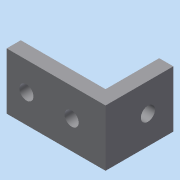
# Autodesk Inventor part: corner bracket
Saved by Autodesk Inventor 2015 (Build 190159000, 159)
## iProperties
Created: 2016-09-09
Part Number: corner bracket
Material: Generic
Document SubType Name: Modeling
Designer: Dustin
Density: 1 g/cm^3
Appearance: Default
Author: Dustin
Autodesk Inventor part; units mm, degrees
ref_plane "YZ Plane" through (0, 0, 0) normal (1, 0, 0) x (0, 1, 0)
ref_plane "XZ Plane" through (0, 0, 0) normal (0, 1, 0) x (-1, 0, 0)
ref_plane "XY Plane" through (0, 0, 0) normal (0, 0, 1) x (1, 0, 0)
sketch "Sketch1" plane through (0, 0, 0) normal (0, 0, 1) x (1, 0, 0)
  line L0 (0, 0) -> (35, 0)
  line L1 (35, 0) -> (35, 5)
  line L2 (35, 5) -> (0, 5)
  line L3 (0, 5) -> (0, 0)
  line L4 (35, 5) -> (30, 5)
  line L5 (30, 5) -> (30, 24)
  line L6 (30, 24) -> (35, 24)
  line L7 (35, 24) -> (35, 5)
  dimension "d0" = 5
  dimension "d1" = 5
  dimension "d2" = 35
  dimension "d3" = 19
  constraints: 16 end point, 4 parallel, 2 horizontal, 2 perpendicular
  measures "d0" distance of L2.end L0.start
  measures "d1" distance of L5.end L6.end
  measures "d2" distance of L0.start L0.end
  measures "d3" distance of L6.end L1.end
extrude "Extrusion1" add sketch "Sketch1" along normal blind 20
sketch "Sketch2" plane through (0, 5, 0) normal (0, 1, 0) x (1, 0, 0)
  line L0 (0, 0) -> (35, 0) projected
  line L1 (0, 0) -> (0, -20) projected
  line L2 (30, 0) -> (30, -20) projected
  point P0 (7, -10)
  point P1 (23, -10)
  dimension "d6" = 10
  dimension "d7" = 7
  dimension "d8" = 7
  measures "d6" distance from line of L0 point (7, -10)
  measures "d7" distance from line of L1 point (7, -10)
  measures "d8" distance from line of L2 point (23, -10)
hole "Hole1" at (7, 5, 10) at (23, 5, 10) direction (0, -1, 0) diameter 5 depth 8 tip angle 118
sketch "Sketch3" plane through (30, 5, 0) normal (-1, 0, 0) x (0, 0, 1)
  line L0 (0, 19) -> (20, 19) projected
  line L1 (0, -5) -> (0, 19) projected
  line L2 (7.5, 0) -> (12.5, 0) projected
  line L3 (20, 19) -> (20, 0) projected
  point P0 (10, 10)
  dimension "d18" = 10
  dimension "d19" = 10
  measures "d18" distance from line of L2 point (10, 10)
  measures "d19" distance from line of L3 point (10, 10)
hole "Hole2" at (30, 15, 10) direction (1, 0, 0) diameter 5 depth 8 tip angle 118
body "Solid1"
